Autodesk Fusion 360 part; units mm, degrees
(part 2 of 2)
equation "d111 = Screw_Dia"
equation "d112 = Screw_Dia + Wall_Thickness * 2"
equation "d113 = -Wall_Thickness"
equation "Screw_Standoff_Height_Above = Ctrl_Height - 2 * Wall_Thickness - Screw_Standoff_Height_Below - Board_PCB_Thickness"
equation "d116 = -Screw_Standoff_Height_Above"
equation "d122 = ShoBtn_l1"
equation "ShoBtn_l1 = 25 mm"
equation "ShoBtn_l2 = 5 mm"
equation "d125 = ShoBtn_l2"
equation "d126 = Wall_Thickness"
equation "d127 = ShoBtn_l2 + Wall_Thickness"
equation "d128 = Wall_Thickness"
equation "d129 = -Wall_Thickness"
equation "ShoSw_Height = 5 mm"
equation "ShoSw_Width = 6 mm"
equation "d143 = -Ctrl_Height + USB_Port_Height"
equation "d148 = micrp_Length"
equation "d149 = micro_Width"
equation "d151 = tolerance_ShoSw"
equation "tolerance_ShoSw = 0.25 mm"
equation "d153 = tolerance_ShoSw"
equation "d154 = tolerance_ShoSw"
equation "d156 = tolerance_ShoSw * 2"
equation "d157 = Wall_Thickness"
equation "d159 = -ShoSw_Height"
equation "d164 = tolerance_ShoSw * 2"
equation "d166 = Ctrl_Height - USB_Port_Height - Wall_Thickness - tolerance_ShoSw * 2"
equation "d172 = -ShoBtn_l1"
equation "d174 = micro_USB_width"
equation "micro_USB_height = 3 mm"
equation "micro_USB_width = 8.5 mm"
equation "ser_Port_Height = 2.7 mm"
equation "ser_Port_Width = 10.2 mm"
equation "d179 = micro_USB_height"
equation "d182 = ser_Port_Height"
equation "d183 = ser_Port_Width"
equation "d184 = ser_Port_Width / 2"
equation "d185 = -Wall_Thickness"
equation "micro_USB_Depth = 1.45 mm"
equation "d190 = d188"
equation "d191 = d188"
equation "d192 = d188"
equation "d197 = -Wall_Thickness + micro_USB_Depth"
equation "d199 = Wall_Thickness - micro_USB_Depth"
equation "d205 = ser_Port_Width"
equation "d207 = Button_ModeSet_Height"
equation "Button_ModeSet_Height = 7 mm" comment "ohne pcb"
equation "Button_ModeSet_cap_height = Ctrl_Height - Wall_Thickness - Screw_Standoff_Height_Below - Button_ModeSet_Height + Button_SetMode_Cap_visHeight"
equation "d213 = Button_ModeSet_cap_height - Wall_Thickness"
equation "Button_SetMode_Cap_visHeight = 1.5 mm"
equation "d216 = Button_ModeSet_cap_height - Wall_Thickness - Button_SetMode_Cap_visHeight - Wall_Thickness"
equation "d220 = -7 mm - Wall_Thickness"
equation "d227 = Wall_Thickness"
equation "d232 = Wall_Thickness"
equation "d234 = Wall_Thickness"
equation "d236 = Wall_Thickness"
equation "LED_Dia = 5.6 mm"
equation "LED_Height = 8.6 mm"
equation "d240 = LED_Dia"
equation "d242 = -LED_Height - Wall_Thickness"
equation "d244 = -Wall_Thickness + 1 mm"
equation "d246 = Wall_Thickness - 1 mm"
equation "d248 = -tolerance_ShoSw"
equation "d249 = -tolerance_ShoSw"
equation "micro_Thickness = 1.55 mm"
equation "d251 = 2 * Wall_Thickness + Screw_Standoff_Height_Below + Board_PCB_Thickness"
equation "d253 = Wall_Thickness + Screw_Standoff_Height_Below"
equation "d255 = -Screw_Standoff_Height_Above - Wall_Thickness"
equation "d257 = Screw_Head_Dia"
equation "d258 = Screw_Dia + 0.5 mm"
equation "d262 = d257 / 2 + 2.5 mm"
equation "d263 = USB_Port_Height"
equation "d265 = Screw_Standoff_Height_Below"
equation "d267 = -Wall_Thickness"
equation "micro_Width = 18 mm"
equation "micrp_Length = 33.2 mm"
equation "d274 = d273 / 2"
equation "d276 = -Ctrl_Height + USB_Port_Height + micro_USB_height + micro_Thickness"
equation "d278 = -Ctrl_Height + USB_Port_Height + micro_USB_height"
named bodies: "Controller Unterseite", "Board", "Controller Oberseite", "Schultertaste L", "Schultertaste R", "Taster Set", "Taster Mode"
